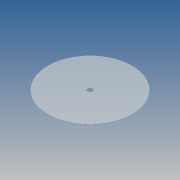
# Autodesk Inventor part: feed-backplane surface
Saved by Autodesk Inventor 2013 SP2 (Build 170200200, 200)
## iProperties
Company: HERA Project
Created: 2013-05-29
Part Number: feed-backplane surface
Material: Glass
Document SubType Name: Modeling
Designer: David DeBoer
Density: 2.18 g/cm^3
Description: Feed backplane conducting surface
Mass: 13748.1 g
Surface Area: 49799.2 cm^2
Volume: 6306.48 cm^3
Author: David DeBoer
Title: Feed backplane surface
Autodesk Inventor part; units mm, degrees
ref_plane "YZ Plane" through (0, 0, 0) normal (1, 0, 0) x (0, 1, 0)
ref_plane "XZ Plane" through (0, 0, 0) normal (0, 1, 0) x (-1, 0, 0)
ref_plane "XY Plane" through (0, 0, 0) normal (0, 0, 1) x (1, 0, 0)
sketch "Sketch1" plane through (0, 0, 0) normal (0, 1, 0) x (-1, 0, 0)
  circle A0 centre (0.5896, 0.4606) radius 736.6
  point P0 (0, 0)
  dimension "d0" = 1473.2
  constraints: 1 centre point
  measures "d0" diameter of A0
extrude "Extrusion1" add sketch "Sketch1" along normal blind 2.54
sketch "Sketch2" plane through (-0.5896, 2.54, 0.4606) normal (0, 1, 0) x (1, 0, 0)
  circle A0 centre (0.5896, 0.4606) radius 44.45
  dimension "d7" = 88.9
  constraints: 1 centre point, 1 coincident
  measures "d7" diameter of A0
extrude "Extrusion2" cut sketch "Sketch2" against normal blind 25.4
body "Solid1"
